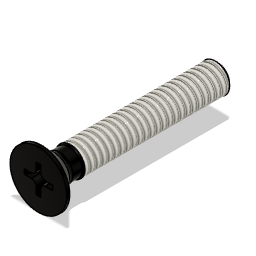
full (Autodesk Fusion 360 archive; units mm, degrees)
design "Countersunk Screw JIS B 1111 - M2x12 - H Steel 4.6 Black"
description: Countersunk Screw JIS B 1111 - M2x12 - H
Autodesk Fusion 360 part; units mm, degrees
sketch "Sketch1" plane through (0, 0, 0) normal (0, 1, 0) x (1, 0, 0)
  line L0 (0, -2.1) -> (-1.9, -2.1)
  line L1 (-1.9, -2.1) -> (-1.9, -1.9)
  line L2 (-1.9, -1.9) -> (-0.9, -0.9)
  line L3 (-1, 0.1) -> (-1, 9.9)
  line L4 (-0.9, -0.9) -> (0, 0) construction
  line L5 (-1, 9.9) -> (0, 9.9)
  line L6 (0, 9.9) -> (0, -2.1)
  line L7 (-0.9, -0.0732) -> (-0.9, -0.9)
  line L8 (-1, 0.1) -> (-0.9, -0.0732)
  dimension "d5" = 45
  dimension "d9" = 2
  dimension "d10" = 12
  dimension "d11" = 3.8
  dimension "d71" = 1.2
  dimension "d72" = 1.8
  dimension "d89" = 9.8
  dimension "d101" = 30
  constraint perpendicular L0 L1
  constraint vertical L3
  constraint perpendicular L3 L5
  constraint collinear L2 L4
  constraint perpendicular L0 L6
  constraint collinear L4.end L0.start L5.end
  constraint coincident L4.end L6
  constraint coincident origin L4
  constraint horizontal L0
  constraint coincident L2.end L4.start
  constraint coincident L7 L8.end
  constraint coincident L7.start L8.end
  measures "d5" angle of L4 L6
  measures "d10" distance of L0.start L5.end
  measures "d71" distance of L0 L2.end
  measures "d89" distance of L5 L3.start
  measures "d101" angle of L3 L8
revolve "Revolve1" add sketch "Sketch1" angle 360 about axis through (0, 0, -9.9) along (0, 0, 1) makes body 1
sketch "Sketch2" plane through (0, 0, 2.1) normal (0, 0, 1) x (1, 0, 0)
  circle A0 centre (0, 0) radius 1.9
  line L0 (-0.1583, 0.95) -> (-0.1583, 0.1583)
  line L1 (-0.1583, 0.1583) -> (-0.95, 0.1583)
  line L2 (0, 0) -> (0, 0.95) construction
  line L3 (0.1583, 0.1583) -> (0.95, 0.1583)
  line L4 (0.1583, 0.95) -> (0.1583, 0.1583)
  line L5 (0.1583, -0.1583) -> (0.95, -0.1583)
  line L6 (0.1583, -0.95) -> (0.1583, -0.1583)
  line L7 (-0.1583, -0.95) -> (-0.1583, -0.1583)
  line L8 (-0.1583, -0.1583) -> (-0.95, -0.1583)
  line L9 (-0.1583, 0.95) -> (0.1583, 0.95)
  line L10 (-0.95, 0.1583) -> (-0.95, -0.1583)
  line L11 (-0.1583, -0.95) -> (0.1583, -0.95)
  line L12 (0.95, -0.1583) -> (0.95, 0.1583)
  line L13 (1.75, 0) -> (22.5, 0)
  dimension "d22" = 0.3167
  dimension "d57" = 1.9
  constraint perpendicular L0 L1
  constraint coincident A0.centre L2.start
  constraint symmetric L0.start L2 L4.start
  constraint symmetric L0.end L2 L3.start
  constraint symmetric L1.end L2 L3.end
  constraint perpendicular L4 L9
  constraint perpendicular L8 L10
  constraint equal L9 L10
  constraint equal L0 L1
  constraint symmetric L1 L8 L13
  constraint horizontal L0.start L2.end
  constraint vertical L2
  constraint symmetric L3 L5 L13
  constraint symmetric L2 L6 L7
  constraint symmetric L9 L11 L13
  constraint collinear L4 L6
  measures "d22" horizontal distance of L0.start L4.start
  measures "d57" distance of L10 L12
extrude "Extrude1" add sketch "Sketch2" against normal blind 1.2 draft -4 separate body contours L0 L1 L3 L4 L5 L6 L7 L8 L9 L10 L11 L12 makes body 2
draft "Draft1" angle -30 neutral plane through (0, 0, 2.1) pull (0, 0, 1) 4 faces at (-0.922, -0.0248, 1.7) (-0.0248, 0.922, 1.7) (0.922, 0.0248, 1.7) (-0.0248, -0.922, 1.7) on bodies 2
fillet "Fillet3" radius 0.3167 4 edges at (-0.1164, 0.1164, 1.5) (0.1164, 0.1164, 1.5) (0.1164, -0.1164, 1.5) (-0.1164, -0.1164, 1.5) on bodies 2
combine "Combine1" operation cut target body 1 tool bodies 2
thread "Thread1" "ISO Metric profile 2.0 M2x0.4 6g" major diameter 1.9335 minor diameter 1.478 pitch 0.4 angle 60 resizes the face on face at (-0.995, 0.0996, -3.3667) on bodies 1
fillet "Fillet5" radius 0.5 1 edges at (-0.8391, 0.3255, 0.9) on bodies 1
sketch "Sketch6" plane through (0, 0, 0) normal (0, 1, 0) x (1, 0, 0)
  line L0 (-0.8, 9.9) -> (-1.02, 9.9)
  line L1 (-1.02, 9.9) -> (-1.02, 9.7)
  line L2 (-1.02, 9.7) -> (-0.8, 9.9)
  line L3 (-1, 9.9) -> (0, 9.9)
  dimension "d102" = 1.02
  dimension "d103" = 0.8
  dimension "d105" = 0.2
  constraint horizontal L0
  constraint perpendicular L0 L1
  constraint coincident L0.start L3
  measures "d102" distance of origin L1
  measures "d103" horizontal distance of origin L0.start
  measures "d105" distance of L0.end L1.end
revolve "Revolve3" cut sketch "Sketch6" angle 360 about axis through (0, 0, 1.75) along (0, 0, 1) bodies 1
equation "d5 = adsk_headang * 0.5"
equation "d9 = adsk_nomdia"
equation "d10 = adsk_nomlen"
equation "d11 = adsk_headdia"
equation "adsk_nomlen = 12.00 mm"
equation "adsk_headh = 1.20 mm"
equation "adsk_headdia = 3.80 mm"
equation "adsk_nomdia = 2.00 mm"
equation "adsk_headang = 90.00 deg"
equation "d22 = adsk_philwidth"
equation "adsk_phildia = 1.90 mm"
equation "d31 = -adsk_phildepth"
equation "adsk_philwidth = adsk_phildia / 6"
equation "adsk_phildepth = 1.20 mm"
equation "d57 = adsk_phildia"
equation "d59 = adsk_philwidth"
equation "d71 = adsk_headh"
equation "d72 = adsk_grpdia"
equation "adsk_grpdia = adsk_nomdia - 0.5 * adsk_pitch1"
equation "d89 = adsk_thrlen"
equation "adsk_thrlen = 9.80 mm"
equation "adsk_pitch1 = 0.40 mm"
equation "adsk_startlen = adsk_nomdia * 0.1"
equation "adsk_headfillet = 0.50 mm"
equation "d96 = adsk_headfillet"
equation "d99 = ( adsk_grpdia / 2 ) * tan(90 deg - adsk_headang / 2) + adsk_headh"
equation "d102 = adsk_nomdia * 0.51"
equation "d103 = adsk_endpointdia / 2"
equation "adsk_endpointdia = adsk_nomdia - adsk_startlen * 2"
equation "d105 = adsk_startlen"
